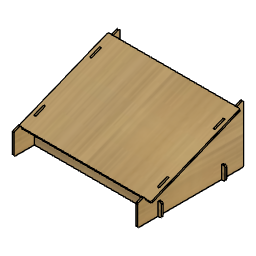
Laptop stand (Autodesk Fusion 360 design; units mm, degrees)
Autodesk Fusion 360 part; units mm, degrees
sketch "Left side" plane through (0, 0, 0) normal (1, 0, 0) x (0, 1, 0) in component "Leg"
  line L0 (0, 0) -> (250, 0)
  line L1 (250, 0) -> (250, 137.5)
  line L2 (250, 137.5) -> (20.2662, 44.6815)
  line L3 (20.2662, 44.6815) -> (15.575, 56.2927)
  line L4 (15.575, 56.2927) -> (0, 50)
  line L5 (0, 50) -> (0, 0)
  line L6 (20.2662, 44.6815) -> (250, 137.5)
  dimension "d2" = 250
  dimension "d4" = 137.5
  dimension "d6" = 50
  dimension "d7" = 22
  dimension "d9" = 15.575
  dimension "d46" = 90
  constraint coincident L0.start L5.end
  constraint horizontal L0
  constraint perpendicular L0 L1
  constraint perpendicular L0 L5
  constraint parallel L2 L4
  measures "d2" distance of L0.start L0.end
  measures "d4" distance of L0.end L1.end
  measures "d6" distance of L4.end L0.start
  measures "d7" angle of L0 L2
  measures "d9" horizontal distance of L3.end L4.end
  measures "d46" angle of L2 L3
extrude "Extrude1" add sketch "Left side" along normal blind 4 makes body 1 in component "Leg"
fillet "Fillet1" radius 3 6 edges at (2, 250, 137.5) (2, 15.575, 56.2927) (2, 0, 50) (2, 20.2662, 44.6815) (2, 0, 0) (2, 250, 0) on bodies 1 in component "Leg"
sketch "Table" plane through (52.5, -12.6752, 31.3723) normal (0, -0.374607, 0.927184) x (1, 0, 0) in component "Table"
  line L0 (-344, 38.5285) -> (-340, 38.5285)
  line L1 (-340, 38.5285) -> (-340, 278.8567)
  line L2 (-340, 278.8567) -> (-344, 278.8567)
  line L3 (-344, 278.8567) -> (-344, 38.5285)
  line L4 (-52.5, 38.5285) -> (-48.5, 38.5285)
  line L5 (-48.5, 38.5285) -> (-48.5, 278.8567)
  line L6 (-48.5, 278.8567) -> (-52.5, 278.8567)
  line L7 (-52.5, 278.8567) -> (-52.5, 38.5285)
  line L8 (-352, 265.6988) -> (-40.5, 265.6988)
  line L9 (-40.5, 265.6988) -> (-40.5, 38.5285)
  line L10 (-40.5, 38.5285) -> (-352, 38.5285)
  line L11 (-352, 38.5285) -> (-352, 265.6988)
  line L12 (-52.5, 235.7228) -> (-48.5, 235.7228)
  line L13 (-48.5, 235.7228) -> (-48.5, 210.7228)
  line L14 (-48.5, 210.7228) -> (-52.5, 210.7228)
  line L15 (-52.5, 210.7228) -> (-52.5, 235.7228)
  line L16 (-196.25, 265.6988) -> (-196.25, 38.5285) construction
  line L17 (-352, 152.1137) -> (-40.5, 152.1137) construction
  line L18 (-340, 235.7228) -> (-344, 235.7228)
  line L19 (-340, 210.7228) -> (-340, 235.7228)
  line L20 (-344, 235.7228) -> (-344, 210.7228)
  line L21 (-344, 210.7228) -> (-340, 210.7228)
  line L22 (-340, 93.5045) -> (-340, 68.5045)
  line L23 (-344, 68.5045) -> (-344, 93.5045)
  line L24 (-340, 68.5045) -> (-344, 68.5045)
  line L25 (-344, 93.5045) -> (-340, 93.5045)
  line L26 (-48.5, 93.5045) -> (-52.5, 93.5045)
  line L27 (-52.5, 93.5045) -> (-52.5, 68.5045)
  line L28 (-48.5, 68.5045) -> (-48.5, 93.5045)
  line L29 (-52.5, 68.5045) -> (-48.5, 68.5045)
  dimension "d22" = 13.1579
  dimension "d23" = 8
  dimension "d24" = 8
  dimension "d25" = 25
  dimension "d26" = 29.976
  constraint horizontal L8
  constraint vertical L9
  constraint horizontal L10
  constraint vertical L11
  constraint collinear L4 L10
  constraint horizontal L12
  constraint vertical L13
  constraint horizontal L14
  constraint vertical L15
  constraint coincident L5 L13.end
  constraint coincident L7 L12.start
  constraint midpoint L8 L16.start
  constraint midpoint L10 L16.end
  constraint midpoint L11 L17.start
  constraint midpoint L9 L17.end
  constraint symmetric L12.start L16 L18.start
  constraint symmetric L12.end L16 L18.end
  constraint symmetric L13.end L16 L20.end
  constraint symmetric L14.end L16 L19.start
  constraint symmetric L12.start L17 L27.end
  constraint symmetric L12.end L17 L28.start
  constraint symmetric L13.end L17 L26.start
  constraint symmetric L14.end L17 L26.end
  constraint symmetric L17 L20.end L23.end
  constraint symmetric L17 L19.start L22.start
  constraint symmetric L17 L18.end L23.start
  constraint symmetric L17 L18.start L22.end
  measures "d22" distance of L6 L8
  measures "d23" distance of L5 L9
  measures "d24" distance of L3 L11
  measures "d25" distance of L12 L14
  measures "d26" distance of L8 L12
extrude "Extrude1'" add sketch "Table" against normal blind 4 separate body contours L0 L1 L3 L10 L24 | L3 L8 L10 L11 L20 L23 | L1 L7 L8 L10 L15 L19 L22 L27 | L4 L5 L7 L10 L29 | L1 L3 L21 L25 | L5 L8 L9 L10 L13 L28 | L1 L3 L8 L18 | L5 L7 L14 L26 | L5 L7 L8 L12 makes body 2 in component "Table"
combine "Combine1" operation cut target body 1 tool bodies 2 keep tools in component "Leg"
fillet "Fillet1'" radius 3 4 edges at (12, 23.797, 43.951) (12, 234.4256, 129.0505) (-299.5, 23.797, 43.951) (-299.5, 234.4256, 129.0505) on bodies 2 in component "Table"
ref_plane "WorkPlane1" through (2, 200, 68.0262) normal (0, 1, 0) x (0, 0, 1) in component "Support"
sketch "Sketch1" plane through (2, 200, 61.1512) normal (0, 1, 0) x (1, 0, 0) in component "Support"
  line L0 (-293.5, -56.1475) -> (-289.5, -56.1475)
  line L1 (-289.5, -56.1475) -> (-289.5, 61.1512)
  line L2 (-289.5, 61.1512) -> (-293.5, 61.1512)
  line L3 (-293.5, 61.1512) -> (-293.5, -56.1475)
  line L4 (-2, -56.1475) -> (2, -56.1475)
  line L5 (2, -56.1475) -> (2, 61.1512)
  line L6 (2, 61.1512) -> (-2, 61.1512)
  line L7 (-2, 61.1512) -> (-2, -56.1475)
  line L8 (10, 61.1512) -> (-301.5, 61.1512)
  line L9 (-301.5, 61.1512) -> (-301.5, 29.9012)
  line L10 (-301.5, 29.9012) -> (10, 29.9012)
  line L11 (10, 29.9012) -> (10, 61.1512)
  line L12 (-301.5, 17.9307) -> (-301.5, -64.9211)
  line L13 (10, -64.9211) -> (10, 17.9307)
  line L14 (10, 45.5262) -> (-301.5, 45.5262)
  dimension "d33" = 31.25
  constraint horizontal L8
  constraint vertical L9
  constraint horizontal L10
  constraint vertical L11
  constraint collinear L2 L8
  constraint collinear L9 L12
  constraint collinear L11 L13
  constraint midpoint L11 L14.start
  constraint midpoint L9 L14.end
  measures "d33" distance of L8 L10
extrude "Extrude1''" add sketch "Sketch1" along normal mid plane 4 separate body contours L3 L9 L10 L14 | L1 L7 L10 L14 | L3 L8 L9 L14 | L1 L2 L3 L8 L14 | L1 L7 L8 L14 | L5 L6 L7 L8 L14 | L5 L10 L11 L14 | L5 L8 L11 L14 makes body 3 in component "Support"
ref_plane "WorkPlane2" through (2, 125, 68.0262) normal (0, 1, 0) x (0, 0, 1) in component "Support"
fillet "Fillet1''" radius 3 4 edges at (12, 200, 31.25) (12, 200, 0) (-299.5, 200, 31.25) (-299.5, 200, 0) on bodies 3 in component "Support"
fillet "Fillet2" radius 0.5 4 edges at (4, 200, 31.25) (0, 200, 31.25) (-287.5, 200, 31.25) (-291.5, 200, 31.25) on bodies 3 in component "Support"
mirror "Mirror1" about plane through (2, 125, 68.0262) normal (0, 1, 0) of bodies 3 makes body 4 in component "Support"
combine "Combine2" operation cut target body 1 tool bodies 4 3 keep tools in component "Leg"
fillet "Fillet2'" radius 0.5 10 edges at (2, 198, 0) (2, 202, 0) (2, 52, 0) (2, 48, 0) (2, 23.0478, 45.8053) (2, 74.0207, 66.3997) (2, 205.8831, 119.6756) (2, 233.6764, 130.9048) (2, 50.8411, 57.0346) (2, 182.7035, 110.3105) on bodies 1 in component "Leg"
sketch "Leg DXF" plane through (4, 0, 0) normal (1, 0, 0) x (0, 1, 0)
  arc A0 (183.1671, 110.4978) -> (182.8908, 109.8469) centre (183.3544, 110.0342) ccw
  line L0 (182.8908, 109.8469) -> (184.2019, 106.6017)
  line L1 (184.2019, 106.6017) -> (75.5191, 62.691)
  line L2 (75.5191, 62.691) -> (74.208, 65.9361)
  arc A1 (74.208, 65.9361) -> (73.5571, 66.2124) centre (73.7444, 65.7488) ccw
  line L3 (73.5571, 66.2124) -> (51.3046, 57.2219)
  arc A2 (51.3046, 57.2219) -> (51.0284, 56.571) centre (51.4919, 56.7583) ccw
  line L4 (51.0284, 56.571) -> (52.3395, 53.3258)
  line L5 (52.3395, 53.3258) -> (24.5462, 42.0966)
  line L6 (24.5462, 42.0966) -> (23.2216, 45.375)
  arc A3 (23.2216, 45.375) -> (22.6389, 45.6733) centre (22.758, 45.1877) ccw
  arc A4 (19.1424, 47.4631) -> (22.6389, 45.6733) centre (21.924, 48.5869) ccw
  line L7 (19.1424, 47.4631) -> (16.6988, 53.5112)
  arc A5 (16.6988, 53.5112) -> (12.7934, 55.1689) centre (13.9173, 52.3873) ccw
  line L8 (12.7934, 55.1689) -> (1.8762, 50.758)
  arc A6 (1.8762, 50.758) -> (0, 47.9765) centre (3, 47.9765) ccw
  line L9 (0, 47.9765) -> (0, 3)
  arc A7 (0, 3) -> (3, 0) centre (3, 3) ccw
  line L10 (3, 0) -> (47.5, 0)
  arc A8 (47.5, 0) -> (48, 0.5) centre (47.5, 0.5) ccw
  line L11 (48, 0.5) -> (48, 15.625)
  line L12 (48, 15.625) -> (52, 15.625)
  line L13 (52, 15.625) -> (52, 0.5)
  arc A9 (52, 0.5) -> (52.5, 0) centre (52.5, 0.5) ccw
  line L14 (52.5, 0) -> (197.5, 0)
  arc A10 (197.5, 0) -> (198, 0.5) centre (197.5, 0.5) ccw
  line L15 (198, 0.5) -> (198, 15.625)
  line L16 (198, 15.625) -> (202, 15.625)
  line L17 (202, 15.625) -> (202, 0.5)
  arc A11 (202, 0.5) -> (202.5, 0) centre (202.5, 0.5) ccw
  line L18 (202.5, 0) -> (247, 0)
  arc A12 (247, 0) -> (250, 3) centre (247, 3) ccw
  line L19 (250, 3) -> (250, 133.0523)
  arc A13 (250, 133.0523) -> (245.8762, 135.8339) centre (247, 133.0523) ccw
  line L20 (245.8762, 135.8339) -> (234.14, 131.0921)
  arc A14 (234.14, 131.0921) -> (233.8637, 130.4412) centre (234.3273, 130.6285) ccw
  line L21 (233.8637, 130.4412) -> (235.1748, 127.1961)
  line L22 (235.1748, 127.1961) -> (207.3815, 115.9669)
  line L23 (207.3815, 115.9669) -> (206.0704, 119.212)
  arc A15 (206.0704, 119.212) -> (205.4195, 119.4883) centre (205.6068, 119.0247) ccw
  line L24 (205.4195, 119.4883) -> (183.1671, 110.4978)
sketch "Table DXF" plane through (0, -12.6752, 31.3723) normal (0, -0.374607, 0.927184) x (1, 0, 0)
  arc A0 (-296.5, 265.6988) -> (-299.5, 262.6988) centre (-296.5, 262.6988) ccw
  line L0 (-299.5, 262.6988) -> (-299.5, 41.5285)
  arc A1 (-299.5, 41.5285) -> (-296.5, 38.5285) centre (-296.5, 41.5285) ccw
  line L1 (-296.5, 38.5285) -> (9, 38.5285)
  arc A2 (9, 38.5285) -> (12, 41.5285) centre (9, 41.5285) ccw
  line L2 (12, 41.5285) -> (12, 262.6988)
  arc A3 (12, 262.6988) -> (9, 265.6988) centre (9, 262.6988) ccw
  line L3 (9, 265.6988) -> (-296.5, 265.6988)
  line L4 (-287.5, 210.7228) -> (-291.5, 210.7228)
  line L5 (-291.5, 210.7228) -> (-291.5, 235.7228)
  line L6 (-291.5, 235.7228) -> (-287.5, 235.7228)
  line L7 (-287.5, 235.7228) -> (-287.5, 210.7228)
  line L8 (4, 68.5045) -> (0, 68.5045)
  line L9 (0, 68.5045) -> (0, 93.5045)
  line L10 (0, 93.5045) -> (4, 93.5045)
  line L11 (4, 93.5045) -> (4, 68.5045)
  line L12 (-291.5, 68.5045) -> (-291.5, 93.5045)
  line L13 (-291.5, 93.5045) -> (-287.5, 93.5045)
  line L14 (-287.5, 93.5045) -> (-287.5, 68.5045)
  line L15 (-287.5, 68.5045) -> (-291.5, 68.5045)
  line L16 (4, 210.7228) -> (0, 210.7228)
  line L17 (0, 210.7228) -> (0, 235.7228)
  line L18 (0, 235.7228) -> (4, 235.7228)
  line L19 (4, 235.7228) -> (4, 210.7228)
sketch "Support DXF" plane through (0, 48, 0) normal (0, -1, 0) x (1, 0, 0)
  arc A0 (-291.5, 30.75) -> (-292, 31.25) centre (-292, 30.75) ccw
  line L0 (-292, 31.25) -> (-296.5, 31.25)
  arc A1 (-296.5, 31.25) -> (-299.5, 28.25) centre (-296.5, 28.25) ccw
  line L1 (-299.5, 28.25) -> (-299.5, 3)
  arc A2 (-299.5, 3) -> (-296.5, 0) centre (-296.5, 3) ccw
  line L2 (-296.5, 0) -> (9, 0)
  arc A3 (9, 0) -> (12, 3) centre (9, 3) ccw
  line L3 (12, 3) -> (12, 28.25)
  arc A4 (12, 28.25) -> (9, 31.25) centre (9, 28.25) ccw
  line L4 (9, 31.25) -> (4.5, 31.25)
  arc A5 (4.5, 31.25) -> (4, 30.75) centre (4.5, 30.75) ccw
  line L5 (4, 30.75) -> (4, 15.625)
  line L6 (4, 15.625) -> (0, 15.625)
  line L7 (0, 15.625) -> (0, 30.75)
  arc A6 (0, 30.75) -> (-0.5, 31.25) centre (-0.5, 30.75) ccw
  line L8 (-0.5, 31.25) -> (-287, 31.25)
  arc A7 (-287, 31.25) -> (-287.5, 30.75) centre (-287, 30.75) ccw
  line L9 (-287.5, 30.75) -> (-287.5, 15.625)
  line L10 (-287.5, 15.625) -> (-291.5, 15.625)
  line L11 (-291.5, 15.625) -> (-291.5, 30.75)
component "Leg" placed x (1, 0, 0) y (0, 1, 0) z (0, 0, 1) at (0, 0, 0)
component "Leg" placed x (1, 0, 0) y (0, 1, 0) z (0, 0, 1) at (-291.5, 0, 0)
component "Table" placed x (1, 0, 0) y (0, 1, 0) z (0, 0, 1) at (0, 0, 0)
component "Support" placed x (1, 0, 0) y (0, 1, 0) z (0, 0, 1) at (0, 0, 0)
equation "main = 250 mm"
equation "d2 = main"
equation "d4 = hæð"
equation "d6 = frontHæð"
equation "d7 = halli"
equation "halli = 22 deg"
equation "d9 = front"
equation "þykkt = 4 mm"
equation "legBreidd = main * 1.15"
equation "d13 = þykkt"
equation "rúnun = 3 mm"
equation "d17 = rúnun"
equation "d21 = legBreidd"
equation "d22 = extraAtThBack"
equation "d25 = topHoles"
equation "d26 = AboveHoles"
equation "d27 = -þykkt"
equation "d30 = rúnun"
equation "d31 = -( main / 5 )"
equation "supportHeight = main / 8"
equation "d33 = supportHeight"
equation "d34 = þykkt / 2"
equation "rúnunSlide = 0.5 mm"
equation "d40 = rúnun"
equation "d42 = rúnunSlide"
equation "d44 = rúnunSlide"
equation "frontHæð = main * 0.2"
equation "d46 = rettHorn"
equation "rettHorn = 90 deg"
equation "extraAtThBack = main / 19"
equation "AboveHoles = main / 8.34"
equation "topHoles = main / 10"
equation "kerf = 0.207 mm"
equation "hæð = main * 0.55"
equation "front = main * 0.0623"
